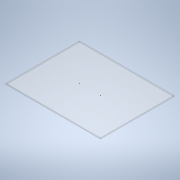
# Autodesk Inventor part: newmiddle
Saved by Autodesk Inventor 2020.1 (Build 241239000, 239)
## iProperties
Created: 2021-08-04
Part Number: newmiddle
Material: PMMA Plastic
Document SubType Name: Modeling
Designer: Caleb
Density: 1.188 g/cm^3
Appearance: Polycarbonate - Clear
Author: Caleb
Autodesk Inventor part; units mm, degrees
ref_plane "YZ Plane" through (0, 0, 0) normal (1, 0, 0) x (0, 1, 0)
ref_plane "XZ Plane" through (0, 0, 0) normal (0, 1, 0) x (-1, 0, 0)
ref_plane "XY Plane" through (0, 0, 0) normal (0, 0, 1) x (1, 0, 0)
sketch "Sketch1" plane through (0, 0, 0) normal (0, 1, 0) x (-1, 0, 0)
  line L0 (-225, 178.8043) -> (225, 178.8043)
  line L1 (225, 178.8043) -> (225, -171.1957)
  line L2 (225, -171.1957) -> (-225, -171.1957)
  line L3 (-225, -171.1957) -> (-225, 178.8043)
  point P0 (0, 0)
  dimension "d14" = 450
  dimension "d15" = 350
  constraints: 8 end point, 2 parallel, 1 horizontal, 1 perpendicular
  measures "d14" distance of L1.end L2.end
  measures "d15" distance between parallel lines of L0 L2
extrude "Extrusion1" add sketch "Sketch1" along normal mid plane 5
sketch "Sketch2" plane through (0, 2.5, 0) normal (0, 1, 0) x (1, 0, 0)
  line L0 (225, 171.1957) -> (-225, 171.1957) projected
  point P0 (0, 0)
  point P1 (-50, -3.8043)
  point P2 (50, -3.8043)
  dimension "d16" = 175
  dimension "d17" = 175
  dimension "d18" = 100
  measures "d16" distance from line of point (50, -3.804) L0
  measures "d17" distance from line of point (-50, -3.804) L0
  measures "d18" distance of point (50, -3.804) point (-50, -3.804)
hole "Hole1" at (-50, 2.5, 3.8043) at (50, 2.5, 3.8043) direction (0, -1, 0) diameter 3 depth 0.5 tip angle 118
body "Solid1"
